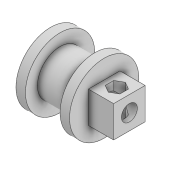
# Autodesk Inventor part: 230307 Bottom Pulley Adjusted
Saved by Autodesk Inventor 2022 (Build 260153000, 153)
## iProperties
Created: 2023-03-07
Part Number: 230307 Bottom Pulley Adjusted
Material: Generic
Document SubType Name: Modeling
Designer: josephinew
Density: 1 g/cm^3
Appearance: Default
Author: josephinew
Autodesk Inventor part; units mm, degrees
ref_plane "YZ Plane" through (0, 0, 0) normal (1, 0, 0) x (0, 1, 0)
ref_plane "XZ Plane" through (0, 0, 0) normal (0, 1, 0) x (-1, 0, 0)
ref_plane "XY Plane" through (0, 0, 0) normal (0, 0, 1) x (1, 0, 0)
sketch "Sketch1" plane through (0, 0, 0) normal (1, 0, 0) x (0, 1, 0)
  circle A0 centre (0, 0) radius 9.144
  line L0 (0, 0) -> (9.144, 0)
  line L1 (9.144, 0) -> (9.144, -9.144)
  line L2 (9.144, -9.144) -> (0, -9.144)
  line L3 (0, -9.144) -> (0, 0)
  line L4 (0, 0) -> (9.144, 0)
  line L5 (9.144, 0) -> (9.144, 9.144)
  line L6 (9.144, 9.144) -> (0, 9.144)
  line L7 (0, 9.144) -> (0, 0)
  dimension "d0" = 18.288
  constraints: 16 end point, 4 parallel, 2 horizontal, 2 perpendicular, 1 centre point, 1 coincident, 1 point on line
  measures "d0" diameter of A0
extrude "Extrusion1" add sketch "Sketch1" along normal blind 13.97
sketch "Sketch5" plane through (13.97, 0, 0) normal (1, 0, 0) x (0, 0, -1)
  line L0 (9.144, 0) -> (9.144, 9.144) projected
  circle A0 centre (0, 0) radius 9.144
  line L1 (9.144, 9.144) -> (-9.144, 9.144)
  line L2 (-9.144, 9.144) -> (-9.144, 0)
  line L3 (-9.144, 0) -> (9.144, 0)
  line L4 (9.144, 0) -> (9.144, 9.144)
  point P0 (0, 9.144)
  constraints: 8 end point, 2 parallel, 2 point on circle, 1 centre point, 1 coincident, 1 horizontal, 1 perpendicular
extrude "Extrusion5" cut sketch "Sketch5" against normal blind 25.4 contours A0 L1 L0 | L2 L1 A0
sketch "Sketch6" plane through (13.97, 0, 0) normal (1, 0, 0) x (0, 0, -1)
  circle A0 centre (0, 0) radius 3.2131
  dimension "d12" = 6.4262
  constraints: 1 centre point, 1 coincident
  measures "d12" diameter of A0
extrude "Extrusion6" cut sketch "Sketch6" against normal blind 25.4
sketch "Sketch7" plane through (0, 0, 0) normal (-1, 0, 0) x (0, 0, 1)
  point P0 (0, 0)
sketch "Sketch8" plane through (13.97, 0, 0) normal (1, 0, 0) x (0, 0, -1)
  circle A0 centre (0, 0) radius 13.97
  dimension "d15" = 27.94
  constraints: 1 centre point, 1 coincident
  measures "d15" diameter of A0
extrude "Extrusion7" add sketch "Sketch8" along normal blind 3.81
sketch "Sketch9" plane through (0, 0, 0) normal (-1, 0, 0) x (0, 0, 1)
  circle A0 centre (0, 0) radius 13.97
  constraints: 1 centre point, 1 coincident
extrude "Extrusion8" add sketch "Sketch9" along normal blind 3.81
sketch "Sketch10" plane through (17.78, 0, 0) normal (1, 0, 0) x (0, 0, -1)
  line L0 (6.35, 0) -> (6.35, 6.35)
  line L1 (6.35, 6.35) -> (0, 6.35)
  line L2 (6.35, 6.35) -> (-6.35, 6.35)
  line L3 (-6.35, 6.35) -> (-6.35, -6.35)
  line L4 (-6.35, -6.35) -> (6.35, -6.35)
  line L5 (6.35, -6.35) -> (6.35, 6.35)
  point P0 (0, 0)
  dimension "d20" = 6.35
  dimension "d21" = 6.35
  dimension "d22" = 12.7
  dimension "d23" = 12.7
  constraints: 12 end point, 2 parallel, 1 horizontal, 1 perpendicular
  measures "d20" distance of L1.end L0.end
  measures "d21" distance of L0.end L0.start
  measures "d22" distance of L4.end L3.end
  measures "d23" distance of L3.end L2.end
extrude "Extrusion9" add sketch "Sketch10" along normal blind 10.16
sketch "Sketch11" plane through (17.78, 6.35, 6.35) normal (0, 1, 0) x (1, 0, 0)
  line L0 (0, 12.7) -> (10.16, 12.7) projected
  line L1 (0, -7.62) -> (0, 20.32) projected
  line L2 (5.08, 3.1902) -> (5.08, 2.9362)
  line L3 (5.08, 9.8043) -> (8.054, 8.0873)
  line L4 (8.054, 8.0873) -> (8.054, 4.6532)
  line L5 (8.054, 4.6532) -> (5.08, 2.9362)
  line L6 (5.08, 2.9362) -> (2.106, 4.6532)
  line L7 (2.106, 4.6532) -> (2.106, 8.0873)
  line L8 (2.106, 8.0873) -> (5.08, 9.8043)
  point P0 (-17.78, 6.35)
  point P1 (-17.78, 7.62)
  point P2 (15.24, 15.24)
  constraints: 14 end point, 1 vertical
extrude "Extrusion10" cut sketch "Sketch11" against normal blind 25.4
sketch "Sketch12" plane through (27.94, 0, 0) normal (1, 0, 0) x (0, 0, -1)
  circle A0 centre (0, 0) radius 3.2131
  constraints: 1 centre point, 1 coincident
extrude "Extrusion11" cut sketch "Sketch12" against normal blind 50.8
body "Solid1"
